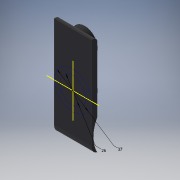
# Autodesk Inventor part: NespressoSpeedfiller-tamper
Saved by Autodesk Inventor 2017 (Build 210142000, 142)
## iProperties
Created: 2018-08-27
Part Number: NespressoSpeedfiller-tamper
Material: Generic
Document SubType Name: Modeling
Designer: 45027374
Density: 1 g/cm^3
Appearance: Default
Author: 45027374
Autodesk Inventor part; units mm, degrees
ref_plane "YZ Plane" through (0, 0, 0) normal (1, 0, 0) x (0, 1, 0)
ref_plane "XZ Plane" through (0, 0, 0) normal (0, 1, 0) x (-1, 0, 0)
ref_plane "XY Plane" through (0, 0, 0) normal (0, 0, 1) x (1, 0, 0)
sketch "Sketch1" plane through (0, 0, 0) normal (0, 1, 0) x (-1, 0, 0)
  line L0 (25.9, 0) -> (-25.9, 0) projected
  line L1 (0, -25.9) -> (0, 25.9) projected
  circle A0 centre (0, 0) radius 18.5 construction
  circle A1 centre (0, 0) radius 13 construction
  dimension "d0" = 37
  dimension "d1" = 26
  constraints: 2 centre point, 2 coincident
  measures "d0" diameter of A0
  measures "d1" diameter of A1
sketch "Sketch2" plane through (0, 0, 0) normal (0, 1, 0) x (-1, 0, 0)
  line L0 (25.9, 0) -> (-25.9, 0) projected
  line L1 (0, -35.8) -> (0, 67.8) projected
  line L2 (-18.5, 53) -> (-18.5, -21)
  line L3 (-18.5, -21) -> (18.5, -21)
  line L4 (18.5, -21) -> (18.5, 53)
  line L5 (-18.5, 53) -> (18.5, 53)
  point P0 (0, 0)
  dimension "d3" = 37
  dimension "d29" = 21
  dimension "d30" = 53
  constraints: 8 end point, 1 horizontal, 1 parallel, 1 other
  measures "d3" distance of L2.end L3.end
  measures "d29" distance between parallel lines of L0 L3
  measures "d30" distance between parallel lines of L5 L0
extrude "Extrusion1" add sketch "Sketch2" along normal blind 6
sketch "Sketch6" plane through (0, 0, 0) normal (0, 1, 0) x (-1, 0, 0)
  line L0 (18.5, -21) -> (-18.5, -21) projected
  line L1 (18.5, 53) -> (18.5, -21) projected
  line L2 (-18.5, -21) -> (18.5, -21)
  line L3 (18.5, -21) -> (18.5, 53)
  line L4 (-18.5, 53) -> (-18.5, -21)
  line L5 (25.9, 0) -> (-25.9, 0) projected
  line L6 (0, -36.3) -> (0, 70.8) projected
  arc A0 (-16, 0) -> (16, 0) centre (0, 0) ccw
  line L7 (16, 0) -> (16, 53)
  line L8 (18.5, 53) -> (-18.5, 53) projected
  line L9 (16, 53) -> (18.5, 53)
  line L10 (-16, 0) -> (-16, 53)
  line L11 (-16, 53) -> (-18.5, 53)
  point P0 (-17.3617, -21)
  dimension "d18" = 32
  constraints: 14 end point, 3 perpendicular, 3 point on line, 2 point on circle, 1 centre point, 1 coincident, 1 collinear, 1 horizontal, 1 parallel, 1 vertical
  measures "d18" diameter of A0
extrude "Extrusion5" [suppressed]
sketch "Sketch4" plane through (0, 0, 0) normal (0, 0, 1) x (1, 0, 0)
  line L0 (-18.5, 0) -> (18.5, 0)
  line L1 (18.5, 0) -> (18.5, -2)
  line L2 (18.5, -2) -> (-18.5, -2)
  line L3 (-18.5, -2) -> (-18.5, 0)
  line L4 (-25.9, 0) -> (25.9, 0) projected
  line L5 (0, -2.4) -> (0, 0.4) projected
  point P0 (0, 0)
  dimension "d10" = 37
  dimension "d11" = 2
  constraints: 8 end point, 2 parallel, 1 collinear, 1 horizontal, 1 perpendicular, 1 other
  measures "d10" distance between parallel lines of L1 L3
  measures "d11" distance of L0.end L1.end
extrude "Extrusion6" [suppressed]
sketch "Sketch5" plane through (0, 0, 0) normal (0, 1, 0) x (-1, 0, 0)
  circle A0 centre (0, 0) radius 18.5 construction
  circle A1 centre (0, 0) radius 18.5 construction
  line L0 (25.9, 0) -> (-25.9, 0) projected
  line L1 (0, -28.9) -> (0, 26.4) projected
  line L2 (-18.5, -21) -> (18.5, -21)
  line L3 (18.5, -21) -> (18.5, -18.5)
  line L4 (18.5, -18.5) -> (-18.5, -18.5)
  line L5 (-18.5, -18.5) -> (-18.5, -21)
  dimension "d25" = 37
  dimension "d26" = 21
  constraints: 8 end point, 2 parallel, 1 centre point, 1 coincident, 1 concentric, 1 horizontal, 1 perpendicular, 1 tangent, 1 other
  measures "d25" distance of L2.start L2.end
  measures "d26" distance between parallel lines of L0 L2
extrude "Extrusion7" [suppressed]
sketch "Sketch7" plane through (0, 0, 0) normal (0, 0, 1) x (1, 0, 0)
  line L0 (-18.5, 0) -> (18.5, 0)
  line L1 (18.5, 0) -> (18.5, -2)
  line L2 (18.5, -2) -> (-18.5, -2)
  line L3 (-18.5, -2) -> (-18.5, 0)
  line L4 (18.5, 0) -> (-18.5, 0) projected
  line L5 (-25.9, 0) -> (25.9, 0) projected
  line L6 (0, -2.4) -> (0, 0.4) projected
  point P0 (-16, 0)
  point P1 (16, 0)
  dimension "d53" = 2
  dimension "d54" = 18.5
  constraints: 8 end point, 2 parallel, 1 collinear, 1 horizontal, 1 perpendicular, 1 other
  measures "d53" distance of L0.end L1.end
  measures "d54" distance between parallel lines of L6 L1
extrude "Extrusion8" [suppressed]
sketch "Sketch8" plane through (0, 0, 0) normal (0, 1, 0) x (-1, 0, 0)
  circle A0 centre (0, 0) radius 12.75
  dimension "d34" = 25.5
  constraints: 1 centre point, 1 coincident
  measures "d34" diameter of A0
extrude "Extrusion9" add sketch "Sketch8" along normal blind 12
pattern_linear "Rectangular Pattern1" count 2 spacing 37 along (0, 0, 1) of "Extrusion9"
sketch "Sketch9" plane through (0, 6, 0) normal (0, 1, 0) x (1, 0, 0)
  circle A0 centre (0, 0) radius 13
  circle A1 centre (0, 0) radius 15
  dimension "d40" = 26
  dimension "d41" = 30
  constraints: 2 centre point, 2 coincident
  measures "d40" diameter of A0
  measures "d41" diameter of A1
extrude "Extrusion10" [suppressed]
sketch "Sketch10" plane through (0, 5, 0) normal (0, 1, 0) x (1, 0, 0)
  arc A0 (16, 0) -> (-16, 0) centre (0, 0) ccw projected
  line L0 (1.5, -18) -> (-1.5, -18)
  line L1 (-29.4, 0) -> (29.4, 0) projected
  line L2 (0, 36.3) -> (0, -70.8) projected
  line L3 (1.5, -12) -> (-1.5, -12)
  line L4 (1.5, -12) -> (1.5, -18)
  line L5 (-1.5, -18) -> (-1.5, -12)
  dimension "d48" = 3
  dimension "d49" = 12
  dimension "d50" = 6
  constraints: 8 end point, 2 perpendicular, 1 horizontal, 1 parallel, 1 other
  measures "d48" distance between parallel lines of L4 L5
  measures "d49" distance between parallel lines of L1 L3
  measures "d50" distance between parallel lines of L0 L3
extrude "Extrusion11" [suppressed]
fillet "Fillet1" radius 5 1 edges at (0, 6, 53)
sketch "Sketch11" plane through (0, 0, 0) normal (0, 1, 0) x (-1, 0, 0)
  line L0 (-18.5, -21) -> (18.5, -21)
  line L1 (18.5, -21) -> (18.5, -47)
  line L2 (18.5, -47) -> (-18.5, -47)
  line L3 (-18.5, -47) -> (-18.5, -21)
  line L4 (25.9, 0) -> (-25.9, 0) projected
  line L5 (0, -60.1) -> (0, 31.6) projected
  point P0 (0, 0)
  dimension "d57" = 26
  dimension "d58" = 21
  dimension "d59" = 37
  constraints: 8 end point, 2 parallel, 1 horizontal, 1 perpendicular, 1 other
  measures "d57" distance of L0.end L1.end
  measures "d58" distance between parallel lines of L4 L0
  measures "d59" distance between parallel lines of L1 L3
extrude "Extrusion12" add sketch "Sketch11" along normal blind 6
sketch "Sketch12" plane through (0, 0, 0) normal (1, 0, 0) x (0, 1, 0)
  line L0 (6, 48) -> (6, -47) projected
  arc A0 (6, -16.5081) -> (5.7334, -47) centre (34, -32) ccw
  line L1 (-6.8, 0) -> (40.8, 0) projected
  line L2 (0, -66.5) -> (0, 70) projected
  line L3 (6, -16.5081) -> (6, -47)
  line L4 (6, -47) -> (5.7334, -47)
  line L5 (0, -47) -> (6, -47) projected
  point P0 (0, 0)
  dimension "d62" = 32
  dimension "d63" = 32
  dimension "d64" = 34
  constraints: 4 end point, 2 point on circle, 2 point on line, 1 centre point, 1 collinear
  measures "d62" radius of A0
  measures "d63" distance from line of L1 A0.centre
  measures "d64" distance from line of A0.centre L2
extrude "Extrusion13" cut sketch "Sketch12" along normal through all both and the other way through all contours L0 L4 A0
fillet "Fillet3" radius 8 1 edges at (0, 0, -47)
body "Solid1"
